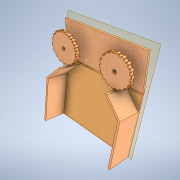
# Autodesk Inventor part: Indexerl
Saved by Autodesk Inventor 2020 (Build 240168000, 168)
## iProperties
Created: 2020-01-22
Part Number: Indexerl
Material: Wood (Birch)
Document SubType Name: Modeling
Designer: JimAndVal
Density: 0.55 g/cm^3
Appearance: Cherry - Natural Low Gloss
Author: JimAndVal
Autodesk Inventor part; units mm, degrees
ref_plane "YZ Plane" through (0, 0, 0) normal (1, 0, 0) x (0, 1, 0)
ref_plane "XZ Plane" through (0, 0, 0) normal (0, 1, 0) x (-1, 0, 0)
ref_plane "XY Plane" through (0, 0, 0) normal (0, 0, 1) x (1, 0, 0)
sketch "Sketch4" plane through (0, 0, 0) normal (0, 0, 1) x (1, 0, 0)
  circle A0 centre (177.8, 0) radius 101.6 construction
  line L0 (271.6029, 16.54) -> (277.8565, 17.6427)
  line L1 (177.8, 0) -> (292.1, 0) construction
  line L2 (267.3057, 32.5774) -> (273.2728, 34.7492)
  line L3 (177.8, 0) -> (292.1, 0) construction
  arc A1 (279.4, 0) -> (277.8565, 17.6427) centre (177.8, 0) ccw
  circle A2 centre (177.8, 0) radius 95.25 construction
  arc A3 (271.6029, 16.54) -> (267.3057, 32.5774) centre (177.8, 0) ccw
  line L4 (260.2889, 47.625) -> (265.7882, 50.8)
  line L5 (250.7657, 61.2255) -> (255.6301, 65.3072)
  arc A4 (273.2728, 34.7492) -> (265.7882, 50.8) centre (177.8, 0) ccw
  arc A5 (260.2889, 47.625) -> (250.7657, 61.2255) centre (177.8, 0) ccw
  line L6 (239.0255, 72.9657) -> (243.1072, 77.8301)
  line L7 (225.425, 82.4889) -> (228.6, 87.9882)
  arc A6 (255.6301, 65.3072) -> (243.1072, 77.8301) centre (177.8, 0) ccw
  arc A7 (239.0255, 72.9657) -> (225.425, 82.4889) centre (177.8, 0) ccw
  line L8 (210.3774, 89.5057) -> (212.5492, 95.4728)
  line L9 (194.34, 93.8029) -> (195.4427, 100.0565)
  arc A8 (228.6, 87.9882) -> (212.5492, 95.4728) centre (177.8, 0) ccw
  arc A9 (210.3774, 89.5057) -> (194.34, 93.8029) centre (177.8, 0) ccw
  line L10 (177.8, 95.25) -> (177.8, 101.6)
  line L11 (161.26, 93.8029) -> (160.1573, 100.0565)
  arc A10 (195.4427, 100.0565) -> (177.8, 101.6) centre (177.8, 0) ccw
  arc A11 (177.8, 95.25) -> (161.26, 93.8029) centre (177.8, 0) ccw
  line L12 (145.2226, 89.5057) -> (143.0508, 95.4728)
  line L13 (130.175, 82.4889) -> (127, 87.9882)
  arc A12 (160.1573, 100.0565) -> (143.0508, 95.4728) centre (177.8, 0) ccw
  arc A13 (145.2226, 89.5057) -> (130.175, 82.4889) centre (177.8, 0) ccw
  line L14 (116.5745, 72.9657) -> (112.4928, 77.8301)
  line L15 (104.8343, 61.2255) -> (99.9699, 65.3072)
  arc A14 (127, 87.9882) -> (112.4928, 77.8301) centre (177.8, 0) ccw
  arc A15 (116.5745, 72.9657) -> (104.8343, 61.2255) centre (177.8, 0) ccw
  line L16 (95.3111, 47.625) -> (89.8118, 50.8)
  line L17 (88.2943, 32.5774) -> (82.3272, 34.7492)
  arc A16 (99.9699, 65.3072) -> (89.8118, 50.8) centre (177.8, 0) ccw
  arc A17 (95.3111, 47.625) -> (88.2943, 32.5774) centre (177.8, 0) ccw
  line L18 (83.9971, 16.54) -> (77.7435, 17.6427)
  line L19 (82.55, 0) -> (76.2, 0)
  arc A18 (82.3272, 34.7492) -> (77.7435, 17.6427) centre (177.8, 0) ccw
  arc A19 (83.9971, 16.54) -> (82.55, 0) centre (177.8, 0) ccw
  line L20 (83.9971, -16.54) -> (77.7435, -17.6427)
  line L21 (88.2943, -32.5774) -> (82.3272, -34.7492)
  arc A20 (76.2, 0) -> (77.7435, -17.6427) centre (177.8, 0) ccw
  arc A21 (83.9971, -16.54) -> (88.2943, -32.5774) centre (177.8, 0) ccw
  line L22 (95.3111, -47.625) -> (89.8118, -50.8)
  line L23 (104.8343, -61.2255) -> (99.9699, -65.3072)
  arc A22 (82.3272, -34.7492) -> (89.8118, -50.8) centre (177.8, 0) ccw
  arc A23 (95.3111, -47.625) -> (104.8343, -61.2255) centre (177.8, 0) ccw
  line L24 (116.5745, -72.9657) -> (112.4928, -77.8301)
  line L25 (130.175, -82.4889) -> (127, -87.9882)
  arc A24 (99.9699, -65.3072) -> (112.4928, -77.8301) centre (177.8, 0) ccw
  arc A25 (116.5745, -72.9657) -> (130.175, -82.4889) centre (177.8, 0) ccw
  line L26 (145.2226, -89.5057) -> (143.0508, -95.4728)
  line L27 (161.26, -93.8029) -> (160.1573, -100.0565)
  arc A26 (127, -87.9882) -> (143.0508, -95.4728) centre (177.8, 0) ccw
  arc A27 (145.2226, -89.5057) -> (161.26, -93.8029) centre (177.8, 0) ccw
  line L28 (177.8, -95.25) -> (177.8, -101.6)
  line L29 (194.34, -93.8029) -> (195.4427, -100.0565)
  arc A28 (160.1573, -100.0565) -> (177.8, -101.6) centre (177.8, 0) ccw
  arc A29 (177.8, -95.25) -> (194.34, -93.8029) centre (177.8, 0) ccw
  line L30 (210.3774, -89.5057) -> (212.5492, -95.4728)
  line L31 (225.425, -82.4889) -> (228.6, -87.9882)
  arc A30 (195.4427, -100.0565) -> (212.5492, -95.4728) centre (177.8, 0) ccw
  arc A31 (210.3774, -89.5057) -> (225.425, -82.4889) centre (177.8, 0) ccw
  line L32 (239.0255, -72.9657) -> (243.1072, -77.8301)
  line L33 (250.7657, -61.2255) -> (255.6301, -65.3072)
  arc A32 (228.6, -87.9882) -> (243.1072, -77.8301) centre (177.8, 0) ccw
  arc A33 (239.0255, -72.9657) -> (250.7657, -61.2255) centre (177.8, 0) ccw
  line L34 (260.2889, -47.625) -> (265.7882, -50.8)
  line L35 (267.3057, -32.5774) -> (273.2728, -34.7492)
  arc A34 (255.6301, -65.3072) -> (265.7882, -50.8) centre (177.8, 0) ccw
  arc A35 (260.2889, -47.625) -> (267.3057, -32.5774) centre (177.8, 0) ccw
  line L36 (271.6029, -16.54) -> (277.8565, -17.6427)
  line L37 (273.05, 0) -> (279.4, 0)
  arc A36 (273.2728, -34.7492) -> (277.8565, -17.6427) centre (177.8, 0) ccw
  arc A37 (271.6029, -16.54) -> (273.05, 0) centre (177.8, 0) ccw
  point P0 (0, 0)
  point P1 (285.2069, 39.0929)
  point P2 (285.2069, 39.0929)
  point P3 (265.3589, 73.4706)
  point P4 (265.3589, 73.4706)
  point P5 (234.95, 98.9867)
  point P6 (234.95, 98.9867)
  point P7 (197.648, 112.5635)
  point P8 (197.648, 112.5635)
  point P9 (157.952, 112.5635)
  point P10 (157.952, 112.5635)
  point P11 (120.65, 98.9867)
  point P12 (120.65, 98.9867)
  point P13 (90.2411, 73.4706)
  point P14 (90.2411, 73.4706)
  point P15 (70.3931, 39.0929)
  point P16 (70.3931, 39.0929)
  point P17 (63.5, 0)
  point P18 (63.5, 0)
  point P19 (70.3931, -39.0929)
  point P20 (70.3931, -39.0929)
  point P21 (90.2411, -73.4706)
  point P22 (90.2411, -73.4706)
  point P23 (120.65, -98.9867)
  point P24 (120.65, -98.9867)
  point P25 (157.952, -112.5635)
  point P26 (157.952, -112.5635)
  point P27 (197.648, -112.5635)
  point P28 (197.648, -112.5635)
  point P29 (234.95, -98.9867)
  point P30 (234.95, -98.9867)
  point P31 (265.3589, -73.4706)
  point P32 (265.3589, -73.4706)
  point P33 (285.2069, -39.0929)
  point P34 (285.2069, -39.0929)
  point P35 (273.2728, -34.7492)
  point P36 (279.4, 0)
  point P37 (255.6301, 65.3072)
  point P38 (228.6, 87.9882)
  point P39 (195.4427, 100.0565)
  point P40 (127, 87.9882)
  point P41 (99.9699, 65.3072)
  point P42 (82.3272, 34.7492)
  point P43 (76.2, 0)
  point P44 (82.3272, -34.7492)
  point P45 (99.9699, -65.3072)
  point P46 (127, -87.9882)
  point P47 (160.1573, -100.0565)
  point P48 (195.4427, -100.0565)
  point P49 (228.6, -87.9882)
  point P50 (255.6301, -65.3072)
  dimension "d21" = 101.6
  dimension "d22" = 10
  dimension "d23" = 101.6
  dimension "d24" = 20
  dimension "d25" = 190.5
  dimension "d28" = 360
  dimension "d71" = 177.8
  constraints: 76 end point, 74 point on circle, 38 centre point, 3 coincident, 2 horizontal, 1 point on line, 235 other
  measures "d21" distance of L1.start L0.end
  measures "d22" angle of L1 L0
  measures "d23" distance of L1.start L2.end
  measures "d24" angle of L3 L2
  measures "d25" diameter of A2
  measures "d71" distance of point (0, 0) L1.start
extrude "Extrusion3" add sketch "Sketch4" along normal mid plane 25.4
fillet "Fillet2" radius 2.54 216 edges at (105.958, -71.842, 12.7) (112.4928, -77.8301, 0) (114.5336, -75.3979, 12.7) (116.5745, -72.9657, 0) (123.1668, -78.0242, 12.7) (130.175, -82.4889, 0) (128.5875, -85.2386, 12.7) (250.7657, 61.2255, 0) (255.8242, 54.6332, 12.7) (194.34, 93.8029, 0) (239.0255, 72.9657, 0) (186.655, 101.2134, 12.7) (202.4525, 92.0044, 12.7) (194.8913, 96.9297, 12.7) (195.4427, 100.0565, 0) (225.425, 82.4889, 0) (253.1979, 63.2664, 12.7) (255.6301, 65.3072, 0) (243.1072, 77.8301, 0) (241.0664, 75.3979, 12.7) (211.4633, 92.4892, 12.7) (212.5492, 95.4728, 0) (227.0125, 85.2386, 12.7) (228.6, 87.9882, 0) (232.4332, 78.0242, 12.7) (249.642, 71.842, 12.7) (220.738, 92.0809, 12.7) (210.3774, 89.5057, 0) (145.2226, -89.5057, 0) (168.945, -101.2134, 12.7) (160.7087, -96.9297, 12.7) (160.1573, -100.0565, 0) (153.1475, -92.0044, 12.7) (143.0508, -95.4728, 0) (144.1367, -92.4892, 12.7) (127, -87.9882, 0) (134.862, -92.0809, 12.7) (161.26, -93.8029, 0) (194.34, -93.8029, 0) (177.8, -95.25, 0) (186.1016, -94.8875, 12.7) (211.4633, -92.4892, 12.7) (212.5492, -95.4728, 0) (204.096, -98.1381, 12.7) (195.4427, -100.0565, 0) (177.8, -101.6, 0) (177.8, -98.425, 12.7) (194.8913, -96.9297, 12.7) (239.0255, -72.9657, 0) (245.1519, -67.3519, 12.7) (241.0664, -75.3979, 12.7) (225.425, -82.4889, 0) (243.1072, -77.8301, 0) (210.3774, -89.5057, 0) (218.0544, -86.3258, 12.7) (227.0125, -85.2386, 12.7) (236.0754, -83.2258, 12.7) (228.6, -87.9882, 0) (267.3057, -32.5774, 0) (270.2892, -33.6633, 12.7) (260.2889, -47.625, 0) (264.1258, -40.2544, 12.7) (263.0386, -49.2125, 12.7) (265.7882, -50.8, 0) (250.7657, -61.2255, 0) (255.6301, -65.3072, 0) (253.1979, -63.2664, 12.7) (261.0258, -58.2754, 12.7) (279.0134, 8.855, 12.7) (273.05, 0, 0) (279.4, 0, 0) (276.225, 0, 12.7) (272.6875, -8.3016, 12.7) (271.6029, -16.54, 0) (274.7297, -17.0913, 12.7) (273.2728, -34.7492, 0) (275.9381, -26.296, 12.7) (277.8565, -17.6427, 0) (260.2889, 47.625, 0) (265.7882, 50.8, 0) (263.0386, 49.2125, 12.7) (269.8809, 42.938, 12.7) (267.3057, 32.5774, 0) (273.2728, 34.7492, 0) (270.2892, 33.6633, 12.7) (271.6029, 16.54, 0) (277.8565, 17.6427, 0) (269.8044, 24.6525, 12.7) (116.5745, 72.9657, 0) (114.5336, 75.3979, 12.7) (112.4928, 77.8301, 0) (104.8343, 61.2255, 0) (110.4481, 67.3519, 12.7) (99.9699, 65.3072, 0) (102.4021, 63.2664, 12.7) (95.3111, 47.625, 0) (94.5742, 58.2754, 12.7) (92.5614, 49.2125, 12.7) (89.8118, 50.8, 0) (91.4742, 40.2544, 12.7) (88.2943, 32.5774, 0) (85.3108, 33.6633, 12.7) (82.3272, 34.7492, 0) (119.5246, 83.2258, 12.7) (274.7297, 17.0913, 12.7) (177.8, 101.6, 0) (130.175, 82.4889, 0) (128.5875, 85.2386, 12.7) (137.5456, 86.3258, 12.7) (145.2226, 89.5057, 0) (143.0508, 95.4728, 0) (144.1367, 92.4892, 12.7) (161.26, 93.8029, 0) (160.1573, 100.0565, 0) (151.504, 98.1381, 12.7) (160.7087, 96.9297, 12.7) (169.4984, 94.8875, 12.7) (177.8, 98.425, 12.7) (177.8, 95.25, 0) (127, 87.9882, 0) (79.6619, 26.296, 12.7) (77.7435, 17.6427, 0) (89.8118, -50.8, 0) (85.7191, -42.938, 12.7) (82.3272, -34.7492, 0) (85.3108, -33.6633, 12.7) (83.9971, -16.54, 0) (85.7956, -24.6525, 12.7) (77.7435, -17.6427, 0) (80.8703, -17.0913, 12.7) (82.55, 0, 0) (79.375, 0, 12.7) (76.2, 0, 0) (76.5866, -8.855, 12.7) (83.9971, 16.54, 0) (82.9125, 8.3016, 12.7) (80.8703, 17.0913, 12.7) (88.2943, -32.5774, 0) (114.5336, -75.3979, -12.7) (123.1668, -78.0242, -12.7) (128.5875, -85.2386, -12.7) (134.862, -92.0809, -12.7) (144.1367, -92.4892, -12.7) (153.1475, -92.0044, -12.7) (160.7087, -96.9297, -12.7) (168.945, -101.2134, -12.7) (177.8, -98.425, -12.7) (186.1016, -94.8875, -12.7) (194.8913, -96.9297, -12.7) (204.096, -98.1381, -12.7) (211.4633, -92.4892, -12.7) (218.0544, -86.3258, -12.7) (227.0125, -85.2386, -12.7) (236.0754, -83.2258, -12.7) (241.0664, -75.3979, -12.7) (245.1519, -67.3519, -12.7) (253.1979, -63.2664, -12.7) (263.0386, -49.2125, -12.7) (261.0258, -58.2754, -12.7) (104.8343, -61.2255, 0) (99.9699, -65.3072, 0) (102.4021, -63.2664, 12.7) (102.4021, -63.2664, -12.7) (99.7758, -54.6332, 12.7) (99.7758, -54.6332, -12.7) (95.3111, -47.625, 0) (92.5614, -49.2125, 12.7) (92.5614, -49.2125, -12.7) (85.7191, -42.938, -12.7) (85.3108, -33.6633, -12.7) (264.1258, -40.2544, -12.7) (270.2892, -33.6633, -12.7) (275.9381, -26.296, -12.7) (274.7297, -17.0913, -12.7) (272.6875, -8.3016, -12.7) (276.225, 0, -12.7) (274.7297, 17.0913, -12.7) (269.8044, 24.6525, -12.7) (270.2892, 33.6633, -12.7) (269.8809, 42.938, -12.7) (279.0134, 8.855, -12.7) (85.7956, -24.6525, -12.7) (80.8703, -17.0913, -12.7) (76.5866, -8.855, -12.7) (241.0664, 75.3979, -12.7) (263.0386, 49.2125, -12.7) (255.8242, 54.6332, -12.7) (253.1979, 63.2664, -12.7) (249.642, 71.842, -12.7) (232.4332, 78.0242, -12.7) (186.655, 101.2134, -12.7) (202.4525, 92.0044, -12.7) (211.4633, 92.4892, -12.7) (227.0125, 85.2386, -12.7) (220.738, 92.0809, -12.7) (194.8913, 96.9297, -12.7) (137.5456, 86.3258, -12.7) (144.1367, 92.4892, -12.7) (160.7087, 96.9297, -12.7) (169.4984, 94.8875, -12.7) (177.8, 98.425, -12.7) (151.504, 98.1381, -12.7) (92.5614, 49.2125, -12.7) (102.4021, 63.2664, -12.7) (94.5742, 58.2754, -12.7) (110.4481, 67.3519, -12.7) (128.5875, 85.2386, -12.7) (119.5246, 83.2258, -12.7) (114.5336, 75.3979, -12.7) (79.375, 0, -12.7) (82.9125, 8.3016, -12.7) (80.8703, 17.0913, -12.7) (85.3108, 33.6633, -12.7) (79.6619, 26.296, -12.7) (91.4742, 40.2544, -12.7) (105.958, -71.842, -12.7)
sketch "Sketch5" plane through (0, 0, 12.7) normal (0, 0, 1) x (1, 0, 0)
  circle A0 centre (177.8, 0) radius 12.7
  point P0 (0, 0)
  dimension "d33" = 25.4
  dimension "d34" = 177.8
  constraints: 1 centre point
  measures "d33" diameter of A0
  measures "d34" distance of point (0, 0) A0.centre
extrude "Extrusion4" cut sketch "Sketch5" against normal through all
sketch "Sketch6" plane through (0, 0, 12.7) normal (0, 0, 1) x (1, 0, 0)
  circle A0 centre (-177.8, 0) radius 101.6 construction
  line L0 (-83.9971, 16.54) -> (-77.7435, 17.6427)
  line L1 (-177.8, 0) -> (-88.9, 0) construction
  line L2 (-88.2943, 32.5774) -> (-82.3272, 34.7492)
  line L3 (-177.8, 0) -> (-88.9, 0) construction
  arc A1 (-76.2, 0) -> (-77.7435, 17.6427) centre (-177.8, 0) ccw
  circle A2 centre (-177.8, 0) radius 95.25 construction
  arc A3 (-83.9971, 16.54) -> (-88.2943, 32.5774) centre (-177.8, 0) ccw
  line L4 (-95.3111, 47.625) -> (-89.8118, 50.8)
  line L5 (-104.8343, 61.2255) -> (-99.9699, 65.3072)
  arc A4 (-82.3272, 34.7492) -> (-89.8118, 50.8) centre (-177.8, 0) ccw
  arc A5 (-95.3111, 47.625) -> (-104.8343, 61.2255) centre (-177.8, 0) ccw
  line L6 (-116.5745, 72.9657) -> (-112.4928, 77.8301)
  line L7 (-130.175, 82.4889) -> (-127, 87.9882)
  arc A6 (-99.9699, 65.3072) -> (-112.4928, 77.8301) centre (-177.8, 0) ccw
  arc A7 (-116.5745, 72.9657) -> (-130.175, 82.4889) centre (-177.8, 0) ccw
  line L8 (-145.2226, 89.5057) -> (-143.0508, 95.4728)
  line L9 (-161.26, 93.8029) -> (-160.1573, 100.0565)
  arc A8 (-127, 87.9882) -> (-143.0508, 95.4728) centre (-177.8, 0) ccw
  arc A9 (-145.2226, 89.5057) -> (-161.26, 93.8029) centre (-177.8, 0) ccw
  line L10 (-177.8, 95.25) -> (-177.8, 101.6)
  line L11 (-194.34, 93.8029) -> (-195.4427, 100.0565)
  arc A10 (-160.1573, 100.0565) -> (-177.8, 101.6) centre (-177.8, 0) ccw
  arc A11 (-177.8, 95.25) -> (-194.34, 93.8029) centre (-177.8, 0) ccw
  line L12 (-210.3774, 89.5057) -> (-212.5492, 95.4728)
  line L13 (-225.425, 82.4889) -> (-228.6, 87.9882)
  arc A12 (-195.4427, 100.0565) -> (-212.5492, 95.4728) centre (-177.8, 0) ccw
  arc A13 (-210.3774, 89.5057) -> (-225.425, 82.4889) centre (-177.8, 0) ccw
  line L14 (-239.0255, 72.9657) -> (-243.1072, 77.8301)
  line L15 (-250.7657, 61.2255) -> (-255.6301, 65.3072)
  arc A14 (-228.6, 87.9882) -> (-243.1072, 77.8301) centre (-177.8, 0) ccw
  arc A15 (-239.0255, 72.9657) -> (-250.7657, 61.2255) centre (-177.8, 0) ccw
  line L16 (-260.2889, 47.625) -> (-265.7882, 50.8)
  line L17 (-267.3057, 32.5774) -> (-273.2728, 34.7492)
  arc A16 (-255.6301, 65.3072) -> (-265.7882, 50.8) centre (-177.8, 0) ccw
  arc A17 (-260.2889, 47.625) -> (-267.3057, 32.5774) centre (-177.8, 0) ccw
  line L18 (-271.6029, 16.54) -> (-277.8565, 17.6427)
  line L19 (-273.05, 0) -> (-279.4, 0)
  arc A18 (-273.2728, 34.7492) -> (-277.8565, 17.6427) centre (-177.8, 0) ccw
  arc A19 (-271.6029, 16.54) -> (-273.05, 0) centre (-177.8, 0) ccw
  line L20 (-271.6029, -16.54) -> (-277.8565, -17.6427)
  line L21 (-267.3057, -32.5774) -> (-273.2728, -34.7492)
  arc A20 (-279.4, 0) -> (-277.8565, -17.6427) centre (-177.8, 0) ccw
  arc A21 (-271.6029, -16.54) -> (-267.3057, -32.5774) centre (-177.8, 0) ccw
  line L22 (-260.2889, -47.625) -> (-265.7882, -50.8)
  line L23 (-250.7657, -61.2255) -> (-255.6301, -65.3072)
  arc A22 (-273.2728, -34.7492) -> (-265.7882, -50.8) centre (-177.8, 0) ccw
  arc A23 (-260.2889, -47.625) -> (-250.7657, -61.2255) centre (-177.8, 0) ccw
  line L24 (-239.0255, -72.9657) -> (-243.1072, -77.8301)
  line L25 (-225.425, -82.4889) -> (-228.6, -87.9882)
  arc A24 (-255.6301, -65.3072) -> (-243.1072, -77.8301) centre (-177.8, 0) ccw
  arc A25 (-239.0255, -72.9657) -> (-225.425, -82.4889) centre (-177.8, 0) ccw
  line L26 (-210.3774, -89.5057) -> (-212.5492, -95.4728)
  line L27 (-194.34, -93.8029) -> (-195.4427, -100.0565)
  arc A26 (-228.6, -87.9882) -> (-212.5492, -95.4728) centre (-177.8, 0) ccw
  arc A27 (-210.3774, -89.5057) -> (-194.34, -93.8029) centre (-177.8, 0) ccw
  line L28 (-177.8, -95.25) -> (-177.8, -101.6)
  line L29 (-161.26, -93.8029) -> (-160.1573, -100.0565)
  arc A28 (-195.4427, -100.0565) -> (-177.8, -101.6) centre (-177.8, 0) ccw
  arc A29 (-177.8, -95.25) -> (-161.26, -93.8029) centre (-177.8, 0) ccw
  line L30 (-145.2226, -89.5057) -> (-143.0508, -95.4728)
  line L31 (-130.175, -82.4889) -> (-127, -87.9882)
  arc A30 (-160.1573, -100.0565) -> (-143.0508, -95.4728) centre (-177.8, 0) ccw
  arc A31 (-145.2226, -89.5057) -> (-130.175, -82.4889) centre (-177.8, 0) ccw
  line L32 (-116.5745, -72.9657) -> (-112.4928, -77.8301)
  line L33 (-104.8343, -61.2255) -> (-99.9699, -65.3072)
  arc A32 (-127, -87.9882) -> (-112.4928, -77.8301) centre (-177.8, 0) ccw
  arc A33 (-116.5745, -72.9657) -> (-104.8343, -61.2255) centre (-177.8, 0) ccw
  line L34 (-95.3111, -47.625) -> (-89.8118, -50.8)
  line L35 (-88.2943, -32.5774) -> (-82.3272, -34.7492)
  arc A34 (-99.9699, -65.3072) -> (-89.8118, -50.8) centre (-177.8, 0) ccw
  arc A35 (-95.3111, -47.625) -> (-88.2943, -32.5774) centre (-177.8, 0) ccw
  line L36 (-83.9971, -16.54) -> (-77.7435, -17.6427)
  line L37 (-82.55, 0) -> (-76.2, 0)
  arc A36 (-82.3272, -34.7492) -> (-77.7435, -17.6427) centre (-177.8, 0) ccw
  arc A37 (-83.9971, -16.54) -> (-82.55, 0) centre (-177.8, 0) ccw
  circle A38 centre (-177.8, 0) radius 12.7
  point P0 (0, 0)
  point P1 (0, 0)
  point P2 (-94.2613, 30.4056)
  point P3 (-94.2613, 30.4056)
  point P4 (-109.6986, 57.1438)
  point P5 (-109.6986, 57.1438)
  point P6 (-133.35, 76.9897)
  point P7 (-133.35, 76.9897)
  point P8 (-162.3627, 87.5494)
  point P9 (-162.3627, 87.5494)
  point P10 (-193.2373, 87.5494)
  point P11 (-193.2373, 87.5494)
  point P12 (-222.25, 76.9897)
  point P13 (-222.25, 76.9897)
  point P14 (-245.9014, 57.1438)
  point P15 (-245.9014, 57.1438)
  point P16 (-261.3387, 30.4056)
  point P17 (-261.3387, 30.4056)
  point P18 (-266.7, 0)
  point P19 (-266.7, 0)
  point P20 (-261.3387, -30.4056)
  point P21 (-261.3387, -30.4056)
  point P22 (-245.9014, -57.1438)
  point P23 (-245.9014, -57.1438)
  point P24 (-222.25, -76.9897)
  point P25 (-222.25, -76.9897)
  point P26 (-193.2373, -87.5494)
  point P27 (-193.2373, -87.5494)
  point P28 (-162.3627, -87.5494)
  point P29 (-162.3627, -87.5494)
  point P30 (-133.35, -76.9897)
  point P31 (-133.35, -76.9897)
  point P32 (-109.6986, -57.1438)
  point P33 (-109.6986, -57.1438)
  point P34 (-94.2613, -30.4056)
  point P35 (-94.2613, -30.4056)
  point P36 (285.9728, -34.7492)
  point P37 (292.1, 0)
  point P38 (285.9728, 34.7492)
  point P39 (268.3301, 65.3072)
  point P40 (241.3, 87.9882)
  point P41 (208.1427, 100.0565)
  point P42 (172.8573, 100.0565)
  point P43 (139.7, 87.9882)
  point P44 (112.6699, 65.3072)
  point P45 (95.0272, 34.7492)
  point P46 (88.9, 0)
  point P47 (95.0272, -34.7492)
  point P48 (112.6699, -65.3072)
  point P49 (139.7, -87.9882)
  point P50 (172.8573, -100.0565)
  point P51 (208.1427, -100.0565)
  point P52 (241.3, -87.9882)
  point P53 (268.3301, -65.3072)
  point P54 (0, 0)
  point P55 (-127, -87.9882)
  point P56 (-99.9699, -65.3072)
  point P57 (-82.3272, -34.7492)
  point P58 (-76.2, 0)
  point P59 (-82.3272, 34.7492)
  point P60 (-99.9699, 65.3072)
  point P61 (-195.4427, 100.0565)
  point P62 (-228.6, 87.9882)
  point P63 (-255.6301, 65.3072)
  point P64 (-273.2728, 34.7492)
  point P65 (-279.4, 0)
  point P66 (-273.2728, -34.7492)
  point P67 (-255.6301, -65.3072)
  point P68 (-228.6, -87.9882)
  point P69 (-195.4427, -100.0565)
  point P70 (-160.1573, -100.0565)
  dimension "d39" = 177.8
  dimension "d40" = 101.6
  dimension "d41" = 10
  dimension "d42" = 101.6
  dimension "d43" = 20
  dimension "d44" = 190.5
  dimension "d45" = 360
  dimension "d46" = 25.4
  dimension "d72" = 0
  constraints: 76 end point, 74 point on circle, 39 centre point, 4 coincident, 2 horizontal, 1 point on line, 235 other
  measures "d39" distance of point (0, 0) L1.start
  measures "d40" distance of L1.start L0.end
  measures "d41" angle of L1 L0
  measures "d42" distance of L1.start L2.end
  measures "d43" angle of L3 L2
  measures "d44" diameter of A2
  measures "d46" diameter of A38
  measures "d72" distance of L1.start A38.centre
extrude "Extrusion5" add sketch "Sketch6" along normal mid plane 25.4
fillet "Fillet3" radius 2.54 217 edges at (-177.8, 101.6, 12.7) (-160.1573, 100.0565, 12.7) (-177.8, 98.425, 25.4) (-168.945, 101.2134, 25.4) (-160.7087, 96.9297, 25.4) (-177.8, 98.425, 0) (-168.945, 101.2134, 0) (-160.7087, 96.9297, 0) (-204.096, 98.1381, 25.4) (-194.8913, 96.9297, 25.4) (-195.4427, 100.0565, 12.7) (-204.096, 98.1381, 0) (-194.8913, 96.9297, 0) (-190.5, 0, 0) (-95.3111, 47.625, 12.7) (-88.2943, 32.5774, 12.7) (-83.9971, 16.54, 12.7) (-82.3272, 34.7492, 12.7) (-77.7435, 17.6427, 12.7) (-89.8118, 50.8, 12.7) (-105.958, 71.842, 25.4) (-102.4021, 63.2664, 25.4) (-99.7758, 54.6332, 25.4) (-92.5614, 49.2125, 25.4) (-85.7191, 42.938, 25.4) (-85.3108, 33.6633, 25.4) (-80.8703, 17.0913, 25.4) (-76.5866, 8.855, 25.4) (-85.7956, 24.6525, 25.4) (-161.26, 93.8029, 12.7) (-145.2226, 89.5057, 12.7) (-143.0508, 95.4728, 12.7) (-130.175, 82.4889, 12.7) (-127, 87.9882, 12.7) (-104.8343, 61.2255, 12.7) (-112.4928, 77.8301, 12.7) (-99.9699, 65.3072, 12.7) (-116.5745, 72.9657, 12.7) (-153.1475, 92.0044, 25.4) (-144.1367, 92.4892, 25.4) (-128.5875, 85.2386, 25.4) (-134.862, 92.0809, 25.4) (-114.5336, 75.3979, 25.4) (-123.1668, 78.0242, 25.4) (-153.1475, 92.0044, 0) (-144.1367, 92.4892, 0) (-128.5875, 85.2386, 0) (-134.862, 92.0809, 0) (-123.1668, 78.0242, 0) (-114.5336, 75.3979, 0) (-105.958, 71.842, 0) (-102.4021, 63.2664, 0) (-99.7758, 54.6332, 0) (-92.5614, 49.2125, 0) (-85.3108, 33.6633, 0) (-85.7191, 42.938, 0) (-79.375, 0, 25.4) (-82.9125, -8.3016, 25.4) (-80.8703, -17.0913, 25.4) (-85.3108, -33.6633, 25.4) (-79.6619, -26.296, 25.4) (-92.5614, -49.2125, 25.4) (-102.4021, -63.2664, 25.4) (-94.5742, -58.2754, 25.4) (-91.4742, -40.2544, 25.4) (-194.34, 93.8029, 12.7) (-177.8, 95.25, 12.7) (-186.1016, 94.8875, 25.4) (-116.5745, -72.9657, 12.7) (-104.8343, -61.2255, 12.7) (-99.9699, -65.3072, 12.7) (-89.8118, -50.8, 12.7) (-95.3111, -47.625, 12.7) (-88.2943, -32.5774, 12.7) (-82.3272, -34.7492, 12.7) (-77.7435, -17.6427, 12.7) (-119.5246, -83.2258, 0) (-114.5336, -75.3979, 0) (-110.4481, -67.3519, 0) (-102.4021, -63.2664, 0) (-94.5742, -58.2754, 0) (-92.5614, -49.2125, 0) (-91.4742, -40.2544, 0) (-85.3108, -33.6633, 0) (-79.6619, -26.296, 0) (-82.9125, -8.3016, 0) (-80.8703, -17.0913, 0) (-79.375, 0, 0) (-85.7956, 24.6525, 0) (-76.5866, 8.855, 0) (-80.8703, 17.0913, 0) (-225.425, 82.4889, 12.7) (-228.6, 87.9882, 12.7) (-227.0125, 85.2386, 25.4) (-218.0544, 86.3258, 25.4) (-218.0544, 86.3258, 0) (-210.3774, 89.5057, 12.7) (-212.5492, 95.4728, 12.7) (-211.4633, 92.4892, 25.4) (-211.4633, 92.4892, 0) (-186.1016, 94.8875, 0) (-227.0125, 85.2386, 0) (-169.4984, -94.8875, 25.4) (-160.7087, -96.9297, 25.4) (-151.504, -98.1381, 25.4) (-144.1367, -92.4892, 25.4) (-128.5875, -85.2386, 25.4) (-110.4481, -67.3519, 25.4) (-114.5336, -75.3979, 25.4) (-119.5246, -83.2258, 25.4) (-137.5456, -86.3258, 25.4) (-241.0664, -75.3979, 0) (-232.4332, -78.0242, 0) (-227.0125, -85.2386, 0) (-220.738, -92.0809, 0) (-202.4525, -92.0044, 0) (-211.4633, -92.4892, 0) (-194.8913, -96.9297, 0) (-186.655, -101.2134, 0) (-177.8, -98.425, 0) (-169.4984, -94.8875, 0) (-160.7087, -96.9297, 0) (-144.1367, -92.4892, 0) (-151.504, -98.1381, 0) (-137.5456, -86.3258, 0) (-128.5875, -85.2386, 0) (-127, -87.9882, 12.7) (-112.4928, -77.8301, 12.7) (-130.175, -82.4889, 12.7) (-145.2226, -89.5057, 12.7) (-143.0508, -95.4728, 12.7) (-160.1573, -100.0565, 12.7) (-161.26, -93.8029, 12.7) (-177.8, -95.25, 12.7) (-177.8, -101.6, 12.7) (-195.4427, -100.0565, 12.7) (-194.34, -93.8029, 12.7) (-273.05, 0, 12.7) (-82.55, 0, 12.7) (-76.2, 0, 12.7) (-83.9971, -16.54, 12.7) (-271.6029, -16.54, 12.7) (-267.3057, -32.5774, 12.7) (-273.2728, -34.7492, 12.7) (-260.2889, -47.625, 12.7) (-250.7657, -61.2255, 12.7) (-255.6301, -65.3072, 12.7) (-239.0255, -72.9657, 12.7) (-243.1072, -77.8301, 12.7) (-225.425, -82.4889, 12.7) (-228.6, -87.9882, 12.7) (-210.3774, -89.5057, 12.7) (-212.5492, -95.4728, 12.7) (-277.8565, -17.6427, 12.7) (-177.8, -98.425, 25.4) (-249.642, -71.842, 25.4) (-241.0664, -75.3979, 25.4) (-232.4332, -78.0242, 25.4) (-227.0125, -85.2386, 25.4) (-220.738, -92.0809, 25.4) (-202.4525, -92.0044, 25.4) (-194.8913, -96.9297, 25.4) (-186.655, -101.2134, 25.4) (-211.4633, -92.4892, 25.4) (-265.7882, -50.8, 12.7) (-270.2892, 33.6633, 0) (-275.9381, 26.296, 0) (-274.7297, 17.0913, 0) (-276.225, 0, 0) (-274.7297, -17.0913, 0) (-279.0134, -8.855, 0) (-269.8044, -24.6525, 0) (-270.2892, -33.6633, 0) (-272.6875, 8.3016, 0) (-269.8809, -42.938, 0) (-263.0386, -49.2125, 0) (-255.8242, -54.6332, 0) (-253.1979, -63.2664, 0) (-249.642, -71.842, 0) (-276.225, 0, 25.4) (-279.0134, -8.855, 25.4) (-274.7297, -17.0913, 25.4) (-269.8044, -24.6525, 25.4) (-270.2892, -33.6633, 25.4) (-269.8809, -42.938, 25.4) (-255.8242, -54.6332, 25.4) (-253.1979, -63.2664, 25.4) (-263.0386, -49.2125, 25.4) (-260.2889, 47.625, 12.7) (-265.7882, 50.8, 12.7) (-263.0386, 49.2125, 0) (-263.0386, 49.2125, 25.4) (-267.3057, 32.5774, 12.7) (-264.1258, 40.2544, 25.4) (-273.2728, 34.7492, 12.7) (-270.2892, 33.6633, 25.4) (-271.6029, 16.54, 12.7) (-277.8565, 17.6427, 12.7) (-275.9381, 26.296, 25.4) (-274.7297, 17.0913, 25.4) (-272.6875, 8.3016, 25.4) (-264.1258, 40.2544, 0) (-279.4, 0, 12.7) (-261.0258, 58.2754, 25.4) (-261.0258, 58.2754, 0) (-250.7657, 61.2255, 12.7) (-255.6301, 65.3072, 12.7) (-253.1979, 63.2664, 0) (-253.1979, 63.2664, 25.4) (-239.0255, 72.9657, 12.7) (-245.1519, 67.3519, 0) (-243.1072, 77.8301, 12.7) (-241.0664, 75.3979, 25.4) (-241.0664, 75.3979, 0) (-236.0754, 83.2258, 0) (-236.0754, 83.2258, 25.4) (-245.1519, 67.3519, 25.4)
sketch "Sketch7" plane through (0, 0, 25.4) normal (0, 0, 1) x (1, 0, 0)
  line L0 (0, 25.4) -> (0, -152.4)
  arc A0 (0, -152.4) -> (0, 25.4) centre (0, -63.5) ccw
  point P0 (0, 0)
  dimension "d51" = 177.8
  dimension "d52" = 25.4
  constraints: 2 end point, 2 point on circle, 1 centre point, 1 midpoint, 1 vertical
  measures "d51" distance of L0.start L0.end
  measures "d52" distance of point (0, 0) L0.start
revolve "Revolution1" [suppressed]
sketch "Sketch9" plane through (0, 0, 25.4) normal (0, 0, 1) x (1, 0, 0)
  point P0 (0, 0)
sketch "Sketch10" plane through (0, 0, 25.4) normal (0, 0, 1) x (1, 0, 0)
  point P0 (0, 0)
ref_plane "Work Plane1" through (0, 0, -101.6) normal (0, 0, 1) x (1, 0, 0)
sketch "Sketch11" plane through (0, 0, -101.6) normal (0, 0, 1) x (1, 0, 0)
  line L0 (-285.75, 114.3) -> (285.75, 114.3)
  line L1 (285.75, 114.3) -> (285.75, -127)
  line L2 (285.75, -127) -> (-285.75, -127)
  line L3 (-285.75, -127) -> (-285.75, 114.3)
  arc A0 (285.75, -127) -> (285.75, -127) centre (867.1766, -127) ccw
  point P0 (0, 0)
  dimension "d74" = 114.3
  dimension "d75" = 127
  dimension "d76" = 285.75
  dimension "d77" = 285.75
  constraints: 8 end point, 2 perpendicular, 2 point on circle, 1 centre point, 1 horizontal, 1 parallel, 1 point on line, 1 tangent
  measures "d74" distance from line of point (0, 0) L0
  measures "d75" vertical distance of point (0, 0) L2.end
  measures "d76" horizontal distance of point (0, 0) L0.start
  measures "d77" horizontal distance of point (0, 0) L0.end
extrude "Extrusion7" add sketch "Sketch11" along normal blind 12.7 separate body contours L0 L1 L2 L3
ref_plane "Work Plane2" through (-285.75, -127, -88.9) normal (0, 0.1736, 0.9848) x (1, 0, 0)
sketch "Sketch12" plane through (-285.75, -127, -88.9) normal (0, 0.1736, 0.9848) x (1, 0, 0)
  line L0 (1.27, -7.6414) -> (1.27, -420.3871)
  line L1 (1.27, -420.3871) -> (570.23, -420.3871)
  line L2 (570.23, -420.3871) -> (570.23, -7.6414)
  line L3 (570.23, -7.6414) -> (1.27, -7.6414)
  line L4 (285.75, 109.6333) -> (285.75, -615.3091) construction
  dimension "d99" = 284.48
  dimension "d100" = 284.48
  constraints: 10 end point, 3 perpendicular, 2 vertical
  measures "d99" distance from line of L4 L0.end
  measures "d100" distance from line of L4 L1.end
extrude "Extrusion8" add sketch "Sketch12" against normal blind 12.7 bodies 2
sketch "Sketch15" plane through (-285.75, -127, -88.9) normal (0, 0.1736, 0.9848) x (1, 0, 0)
  line L0 (570.23, -7.6414) -> (1.27, -7.6414) construction
  line L1 (285.75, -7.6414) -> (285.75, -316.5947) construction
  line L2 (285.75, -7.6414) -> (120.65, -7.6414) construction
  line L3 (120.65, -7.6414) -> (120.65, -314.2839) construction
  line L4 (120.65, -7.6414) -> (443.7997, -7.6414) construction
  line L5 (1.27, -7.6414) -> (763.27, -7.6414) construction
  line L6 (1.27, -420.3871) -> (570.23, -420.3871) projected
  line L7 (120.65, -7.6414) -> (102.6922, -7.6414)
  line L8 (450.85, -7.6414) -> (450.85, -314.2839) construction
  line L9 (450.85, -7.6414) -> (557.53, -114.3214)
  line L10 (570.23, -109.0636) -> (570.23, -420.3871)
  line L11 (570.23, -420.3871) -> (570.23, -109.0636)
  line L12 (570.23, -420.3871) -> (557.53, -420.3871)
  line L13 (450.85, -7.6414) -> (468.8078, -7.6414)
  line L14 (468.8078, -7.6414) -> (570.23, -109.0636)
  line L15 (557.53, -420.3871) -> (557.53, -114.3214)
  line L16 (1.27, -420.3871) -> (1.27, -109.0636)
  line L17 (1.27, -109.0636) -> (1.27, -420.3871)
  line L18 (13.97, -420.3871) -> (13.97, -114.3214)
  line L19 (1.27, -420.3871) -> (13.97, -420.3871)
  line L20 (102.6922, -7.6414) -> (1.27, -109.0636)
  line L21 (120.65, -7.6414) -> (102.6922, -7.6414)
  line L22 (120.65, -7.6414) -> (120.65, -314.2839) construction
  line L23 (120.65, -7.6414) -> (13.97, -114.3214)
  point P0 (285.75, 109.6333)
  point P1 (127.7003, -7.6414)
  point P2 (1.27, -420.3871)
  point P3 (1.27, -420.3871)
  point P4 (13.97, -420.3871)
  dimension "d102" = 165.1
  dimension "d108" = 17.9578
  constraints: 44 end point, 11 symmetric about line, 2 horizontal, 2 point on line, 1 midpoint, 1 perpendicular, 1 vertical
  measures "d102" distance of L1.start L2.end
  measures "d108" distance of L2.end L7.end
extrude "Extrusion10" add sketch "Sketch15" along normal blind 152.4 bodies 2
body "Solid2"
body "Solid3"
body "Solid4"
